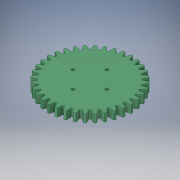
# Autodesk Inventor part: 000.302 - Втулка
Saved by Autodesk Inventor 2019 (Build 230136000, 136)
## iProperties
Created: 2020-02-27
Part Number: 000.302 - Втулка
Material: Пластик АБС
Document SubType Name: Modeling
Designer: Петров Иван
Density: 1.06 g/cm^3
Appearance: Гладкий — темный цвет морской волны
Author: Петров Иван
Autodesk Inventor part; units mm, degrees
ref_plane "YZ Plane" through (0, 0, 0) normal (1, 0, 0) x (0, 1, 0)
ref_plane "XZ Plane" through (0, 0, 0) normal (0, 1, 0) x (-1, 0, 0)
ref_plane "XY Plane" through (0, 0, 0) normal (0, 0, 1) x (1, 0, 0)
sketch "Эскиз1" plane through (0, 0, 0) normal (0, 1, 0) x (-1, 0, 0)
  circle A0 centre (0, 0) radius 12.5
  dimension "d0" = 25
  constraints: 1 centre point, 1 coincident
  measures "d0" diameter of A0
extrude "Выдавливание1" add sketch "Эскиз1" along normal blind 8
sketch "Эскиз2" plane through (0, 8, 0) normal (0, 1, 0) x (1, 0, 0)
  circle A0 centre (0, 0) radius 23
  dimension "d3" = 46
  constraints: 1 centre point, 1 coincident
  measures "d3" diameter of A0
extrude "Выдавливание2" add sketch "Эскиз2" along normal blind 2
sketch "Эскиз3" plane through (0, 10, 0) normal (0, 1, 0) x (1, 0, 0)
  arc A0 (-8.1938, 41.193) -> (-8.7829, 35.8928) centre (15.46, 35.881) ccw
  arc A1 (-8.7829, 35.8928) -> (-10.3402, 35.4755) centre (0, 0) ccw
  arc A2 (-10.3402, 35.4755) -> (-13.5005, 39.7711) centre (-31.3293, 23.3439) ccw
  arc A3 (-13.5005, 39.7711) -> (-15.2224, 39.1443) centre (0, 0) ccw
  arc A4 (-15.2224, 39.1443) -> (-14.8822, 33.8224) centre (8.9945, 38.0205) ccw
  arc A5 (-14.8822, 33.8224) -> (-16.3433, 33.141) centre (0, 0) ccw
  arc A6 (-16.3433, 33.141) -> (-20.2015, 36.8225) centre (-34.9069, 17.549) ccw
  arc A7 (-20.2015, 36.8225) -> (-21.7885, 35.9063) centre (0, 0) ccw
  arc A8 (-21.7885, 35.9063) -> (-20.5293, 30.7243) centre (2.2556, 39.0048) ccw
  arc A9 (-20.5293, 30.7243) -> (-21.8499, 29.7995) centre (0, 0) ccw
  arc A10 (-21.8499, 29.7995) -> (-26.2888, 32.7551) centre (-37.424, 11.2208) ccw
  arc A11 (-26.2888, 32.7551) -> (-27.6925, 31.5773) centre (0, 0) ccw
  arc A12 (-27.6925, 31.5773) -> (-25.5526, 26.6926) centre (-4.5518, 38.8039) ccw
  arc A13 (-25.5526, 26.6926) -> (-26.6926, 25.5526) centre (0, 0) ccw
  arc A14 (-26.6926, 25.5526) -> (-31.5773, 27.6925) centre (-38.8039, 4.5518) ccw
  arc A15 (-31.5773, 27.6925) -> (-32.7551, 26.2888) centre (0, 0) ccw
  arc A16 (-32.7551, 26.2888) -> (-29.7995, 21.8499) centre (-11.2208, 37.424) ccw
  arc A17 (-29.7995, 21.8499) -> (-30.7243, 20.5293) centre (0, 0) ccw
  arc A18 (-30.7243, 20.5293) -> (-35.9063, 21.7885) centre (-39.0048, -2.2556) ccw
  arc A19 (-35.9063, 21.7885) -> (-36.8225, 20.2015) centre (0, 0) ccw
  arc A20 (-36.8225, 20.2015) -> (-33.141, 16.3433) centre (-17.549, 34.9069) ccw
  arc A21 (-33.141, 16.3433) -> (-33.8224, 14.8822) centre (0, 0) ccw
  arc A22 (-33.8224, 14.8822) -> (-39.1443, 15.2224) centre (-38.0205, -8.9945) ccw
  arc A23 (-39.1443, 15.2224) -> (-39.7711, 13.5005) centre (0, 0) ccw
  arc A24 (-39.7711, 13.5005) -> (-35.4755, 10.3402) centre (-23.3439, 31.3293) ccw
  arc A25 (-35.4755, 10.3402) -> (-35.8928, 8.7829) centre (0, 0) ccw
  arc A26 (-35.8928, 8.7829) -> (-41.193, 8.1938) centre (-35.881, -15.46) ccw
  arc A27 (-41.193, 8.1938) -> (-41.5112, 6.3892) centre (0, 0) ccw
  arc A28 (-41.5112, 6.3892) -> (-36.7321, 4.0228) centre (-28.4295, 26.7997) ccw
  arc A29 (-36.7321, 4.0228) -> (-36.8726, 2.4168) centre (0, 0) ccw
  arc A30 (-36.8726, 2.4168) -> (-41.99, 0.9162) centre (-32.6513, -21.4558) ccw
  arc A31 (-41.99, 0.9162) -> (-41.99, -0.9162) centre (0, 0) ccw
  arc A32 (-41.99, -0.9162) -> (-36.8726, -2.4168) centre (-32.6513, 21.4558) ccw
  arc A33 (-36.8726, -2.4168) -> (-36.7321, -4.0228) centre (0, 0) ccw
  arc A34 (-36.7321, -4.0228) -> (-41.5112, -6.3892) centre (-28.4295, -26.7997) ccw
  arc A35 (-41.5112, -6.3892) -> (-41.193, -8.1938) centre (0, 0) ccw
  arc A36 (-41.193, -8.1938) -> (-35.8928, -8.7829) centre (-35.881, 15.46) ccw
  arc A37 (-35.8928, -8.7829) -> (-35.4755, -10.3402) centre (0, 0) ccw
  arc A38 (-35.4755, -10.3402) -> (-39.7711, -13.5005) centre (-23.3439, -31.3293) ccw
  arc A39 (-39.7711, -13.5005) -> (-39.1443, -15.2224) centre (0, 0) ccw
  arc A40 (-39.1443, -15.2224) -> (-33.8224, -14.8822) centre (-38.0205, 8.9945) ccw
  arc A41 (-33.8224, -14.8822) -> (-33.141, -16.3433) centre (0, 0) ccw
  arc A42 (-33.141, -16.3433) -> (-36.8225, -20.2015) centre (-17.549, -34.9069) ccw
  arc A43 (-36.8225, -20.2015) -> (-35.9063, -21.7885) centre (0, 0) ccw
  arc A44 (-35.9063, -21.7885) -> (-30.7243, -20.5293) centre (-39.0048, 2.2556) ccw
  arc A45 (-30.7243, -20.5293) -> (-29.7995, -21.8499) centre (0, 0) ccw
  arc A46 (-29.7995, -21.8499) -> (-32.7551, -26.2888) centre (-11.2208, -37.424) ccw
  arc A47 (-32.7551, -26.2888) -> (-31.5773, -27.6925) centre (0, 0) ccw
  arc A48 (-31.5773, -27.6925) -> (-26.6926, -25.5526) centre (-38.8039, -4.5518) ccw
  arc A49 (-26.6926, -25.5526) -> (-25.5526, -26.6926) centre (0, 0) ccw
  arc A50 (-25.5526, -26.6926) -> (-27.6925, -31.5773) centre (-4.5518, -38.8039) ccw
  arc A51 (-27.6925, -31.5773) -> (-26.2888, -32.7551) centre (0, 0) ccw
  arc A52 (-26.2888, -32.7551) -> (-21.8499, -29.7995) centre (-37.424, -11.2208) ccw
  arc A53 (-21.8499, -29.7995) -> (-20.5293, -30.7243) centre (0, 0) ccw
  arc A54 (-20.5293, -30.7243) -> (-21.7885, -35.9063) centre (2.2556, -39.0048) ccw
  arc A55 (-21.7885, -35.9063) -> (-20.2015, -36.8225) centre (0, 0) ccw
  arc A56 (-20.2015, -36.8225) -> (-16.3433, -33.141) centre (-34.9069, -17.549) ccw
  arc A57 (-16.3433, -33.141) -> (-14.8822, -33.8224) centre (0, 0) ccw
  arc A58 (-14.8822, -33.8224) -> (-15.2224, -39.1443) centre (8.9945, -38.0205) ccw
  arc A59 (-15.2224, -39.1443) -> (-13.5005, -39.7711) centre (0, 0) ccw
  arc A60 (-13.5005, -39.7711) -> (-10.3402, -35.4755) centre (-31.3293, -23.3439) ccw
  arc A61 (-10.3402, -35.4755) -> (-8.7829, -35.8928) centre (0, 0) ccw
  arc A62 (-8.7829, -35.8928) -> (-8.1938, -41.193) centre (15.46, -35.881) ccw
  arc A63 (-8.1938, -41.193) -> (-6.3892, -41.5112) centre (0, 0) ccw
  arc A64 (-6.3892, -41.5112) -> (-4.0228, -36.7321) centre (-26.7997, -28.4295) ccw
  arc A65 (-4.0228, -36.7321) -> (-2.4168, -36.8726) centre (0, 0) ccw
  arc A66 (-2.4168, -36.8726) -> (-0.9162, -41.99) centre (21.4558, -32.6513) ccw
  arc A67 (-0.9162, -41.99) -> (0.9162, -41.99) centre (0, 0) ccw
  arc A68 (0.9162, -41.99) -> (2.4168, -36.8726) centre (-21.4558, -32.6513) ccw
  arc A69 (2.4168, -36.8726) -> (4.0228, -36.7321) centre (0, 0) ccw
  arc A70 (4.0228, -36.7321) -> (6.3892, -41.5112) centre (26.7997, -28.4295) ccw
  arc A71 (6.3892, -41.5112) -> (8.1938, -41.193) centre (0, 0) ccw
  arc A72 (8.1938, -41.193) -> (8.7829, -35.8928) centre (-15.46, -35.881) ccw
  arc A73 (8.7829, -35.8928) -> (10.3402, -35.4755) centre (0, 0) ccw
  arc A74 (10.3402, -35.4755) -> (13.5005, -39.7711) centre (31.3293, -23.3439) ccw
  arc A75 (13.5005, -39.7711) -> (15.2224, -39.1443) centre (0, 0) ccw
  arc A76 (15.2224, -39.1443) -> (14.8822, -33.8224) centre (-8.9945, -38.0205) ccw
  arc A77 (14.8822, -33.8224) -> (16.3433, -33.141) centre (0, 0) ccw
  arc A78 (16.3433, -33.141) -> (20.2015, -36.8225) centre (34.9069, -17.549) ccw
  arc A79 (20.2015, -36.8225) -> (21.7885, -35.9063) centre (0, 0) ccw
  arc A80 (21.7885, -35.9063) -> (20.5293, -30.7243) centre (-2.2556, -39.0048) ccw
  arc A81 (20.5293, -30.7243) -> (21.8499, -29.7995) centre (0, 0) ccw
  arc A82 (21.8499, -29.7995) -> (26.2888, -32.7551) centre (37.424, -11.2208) ccw
  arc A83 (26.2888, -32.7551) -> (27.6925, -31.5773) centre (0, 0) ccw
  arc A84 (27.6925, -31.5773) -> (25.5526, -26.6926) centre (4.5518, -38.8039) ccw
  arc A85 (25.5526, -26.6926) -> (26.6926, -25.5526) centre (0, 0) ccw
  arc A86 (26.6926, -25.5526) -> (31.5773, -27.6925) centre (38.8039, -4.5518) ccw
  arc A87 (31.5773, -27.6925) -> (32.7551, -26.2888) centre (0, 0) ccw
  arc A88 (32.7551, -26.2888) -> (29.7995, -21.8499) centre (11.2208, -37.424) ccw
  arc A89 (29.7995, -21.8499) -> (30.7243, -20.5293) centre (0, 0) ccw
  arc A90 (30.7243, -20.5293) -> (35.9063, -21.7885) centre (39.0048, 2.2556) ccw
  arc A91 (35.9063, -21.7885) -> (36.8225, -20.2015) centre (0, 0) ccw
  arc A92 (36.8225, -20.2015) -> (33.141, -16.3433) centre (17.549, -34.9069) ccw
  arc A93 (33.141, -16.3433) -> (33.8224, -14.8822) centre (0, 0) ccw
  arc A94 (33.8224, -14.8822) -> (39.1443, -15.2224) centre (38.0205, 8.9945) ccw
  arc A95 (39.1443, -15.2224) -> (39.7711, -13.5005) centre (0, 0) ccw
  arc A96 (39.7711, -13.5005) -> (35.4755, -10.3402) centre (23.3439, -31.3293) ccw
  arc A97 (35.4755, -10.3402) -> (35.8928, -8.7829) centre (0, 0) ccw
  arc A98 (35.8928, -8.7829) -> (41.193, -8.1938) centre (35.881, 15.46) ccw
  arc A99 (41.193, -8.1938) -> (41.5112, -6.3892) centre (0, 0) ccw
  arc A100 (41.5112, -6.3892) -> (36.7321, -4.0228) centre (28.4295, -26.7997) ccw
  arc A101 (36.7321, -4.0228) -> (36.8726, -2.4168) centre (0, 0) ccw
  arc A102 (36.8726, -2.4168) -> (41.99, -0.9162) centre (32.6513, 21.4558) ccw
  arc A103 (41.99, -0.9162) -> (41.99, 0.9162) centre (0, 0) ccw
  arc A104 (41.99, 0.9162) -> (36.8726, 2.4168) centre (32.6513, -21.4558) ccw
  arc A105 (36.8726, 2.4168) -> (36.7321, 4.0228) centre (0, 0) ccw
  arc A106 (36.7321, 4.0228) -> (41.5112, 6.3892) centre (28.4295, 26.7997) ccw
  arc A107 (41.5112, 6.3892) -> (41.193, 8.1938) centre (0, 0) ccw
  arc A108 (41.193, 8.1938) -> (35.8928, 8.7829) centre (35.881, -15.46) ccw
  arc A109 (35.8928, 8.7829) -> (35.4755, 10.3402) centre (0, 0) ccw
  arc A110 (35.4755, 10.3402) -> (39.7711, 13.5005) centre (23.3439, 31.3293) ccw
  arc A111 (39.7711, 13.5005) -> (39.1443, 15.2224) centre (0, 0) ccw
  arc A112 (39.1443, 15.2224) -> (33.8224, 14.8822) centre (38.0205, -8.9945) ccw
  arc A113 (33.8224, 14.8822) -> (33.141, 16.3433) centre (0, 0) ccw
  arc A114 (33.141, 16.3433) -> (36.8225, 20.2015) centre (17.549, 34.9069) ccw
  arc A115 (36.8225, 20.2015) -> (35.9063, 21.7885) centre (0, 0) ccw
  arc A116 (35.9063, 21.7885) -> (30.7243, 20.5293) centre (39.0048, -2.2556) ccw
  arc A117 (30.7243, 20.5293) -> (29.7995, 21.8499) centre (0, 0) ccw
  arc A118 (29.7995, 21.8499) -> (32.7551, 26.2888) centre (11.2208, 37.424) ccw
  arc A119 (32.7551, 26.2888) -> (31.5773, 27.6925) centre (0, 0) ccw
  arc A120 (31.5773, 27.6925) -> (26.6926, 25.5526) centre (38.8039, 4.5518) ccw
  arc A121 (26.6926, 25.5526) -> (25.5526, 26.6926) centre (0, 0) ccw
  arc A122 (25.5526, 26.6926) -> (27.6925, 31.5773) centre (4.5518, 38.8039) ccw
  arc A123 (27.6925, 31.5773) -> (26.2888, 32.7551) centre (0, 0) ccw
  arc A124 (26.2888, 32.7551) -> (21.8499, 29.7995) centre (37.424, 11.2208) ccw
  arc A125 (21.8499, 29.7995) -> (20.5293, 30.7243) centre (0, 0) ccw
  arc A126 (20.5293, 30.7243) -> (21.7885, 35.9063) centre (-2.2556, 39.0048) ccw
  arc A127 (21.7885, 35.9063) -> (20.2015, 36.8225) centre (0, 0) ccw
  arc A128 (20.2015, 36.8225) -> (16.3433, 33.141) centre (34.9069, 17.549) ccw
  arc A129 (16.3433, 33.141) -> (14.8822, 33.8224) centre (0, 0) ccw
  arc A130 (14.8822, 33.8224) -> (15.2224, 39.1443) centre (-8.9945, 38.0205) ccw
  arc A131 (15.2224, 39.1443) -> (13.5005, 39.7711) centre (0, 0) ccw
  arc A132 (13.5005, 39.7711) -> (10.3402, 35.4755) centre (31.3293, 23.3439) ccw
  arc A133 (10.3402, 35.4755) -> (8.7829, 35.8928) centre (0, 0) ccw
  arc A134 (8.7829, 35.8928) -> (8.1938, 41.193) centre (-15.46, 35.881) ccw
  arc A135 (8.1938, 41.193) -> (6.3892, 41.5112) centre (0, 0) ccw
  arc A136 (6.3892, 41.5112) -> (4.0228, 36.7321) centre (26.7997, 28.4295) ccw
  arc A137 (4.0228, 36.7321) -> (2.4168, 36.8726) centre (0, 0) ccw
  arc A138 (2.4168, 36.8726) -> (0.9162, 41.99) centre (-21.4558, 32.6513) ccw
  arc A139 (0.9162, 41.99) -> (-0.9162, 41.99) centre (0, 0) ccw
  arc A140 (-0.9162, 41.99) -> (-2.4168, 36.8726) centre (21.4558, 32.6513) ccw
  arc A141 (-2.4168, 36.8726) -> (-4.0228, 36.7321) centre (0, 0) ccw
  arc A142 (-4.0228, 36.7321) -> (-6.3892, 41.5112) centre (-26.7997, 28.4295) ccw
  arc A143 (-6.3892, 41.5112) -> (-8.1938, 41.193) centre (0, 0) ccw
  constraints: 288 point on circle, 144 centre point
extrude "Выдавливание3" add sketch "Эскиз3" along normal blind 8
sketch "Эскиз4" plane through (0, 8, 0) normal (0, -1, 0) x (1, 0, 0)
  line L0 (0, 0) -> (0, -17)
  line L1 (4, -17) -> (2, -20.4641)
  line L2 (2, -20.4641) -> (-2, -20.4641)
  line L3 (-2, -20.4641) -> (-4, -17)
  line L4 (-4, -17) -> (-2, -13.5359)
  line L5 (-2, -13.5359) -> (2, -13.5359)
  line L6 (2, -13.5359) -> (4, -17)
  dimension "d8" = 17
  dimension "d9" = 8
  constraints: 14 end point, 1 coincident, 1 vertical, 13 other
  measures "d8" distance of L0.start L0.end
  measures "d9" distance of L3.end L1.start
extrude "Выдавливание4" cut sketch "Эскиз4" against normal blind 3.3
sketch "Эскиз6" plane through (0, 11.3, 0) normal (0, -1, 0) x (1, 0, 0)
  circle A0 centre (0, 0) radius 12.5 projected
  line L0 (0, 0) -> (0, -17)
  line L1 (3.05, -17) -> (1.525, -19.6414)
  line L2 (1.525, -19.6414) -> (-1.525, -19.6414)
  line L3 (-1.525, -19.6414) -> (-3.05, -17)
  line L4 (-3.05, -17) -> (-1.525, -14.3586)
  line L5 (-1.525, -14.3586) -> (1.525, -14.3586)
  line L6 (1.525, -14.3586) -> (3.05, -17)
  dimension "d16" = 17
  dimension "d17" = 6.1
  constraints: 14 end point, 1 coincident, 1 vertical, 13 other
  measures "d16" distance of L0.start L0.end
  measures "d17" distance of L3.end L1.start
extrude "Выдавливание6" cut sketch "Эскиз6" against normal blind 2.6 contours L1 L2 L3 L4 L5 L6
sketch "Эскиз7" plane through (0, 13.9, 0) normal (0, -1, 0) x (1, 0, 0)
  circle A0 centre (0, 0) radius 12.5 projected
  line L0 (0, 0) -> (0, -17)
  circle A1 centre (0, -17) radius 1.5
  dimension "d20" = 17
  dimension "d21" = 3
  constraints: 2 end point, 1 centre point, 1 coincident, 1 vertical
  measures "d20" distance of L0.start L0.end
  measures "d21" diameter of A1
extrude "Выдавливание7" cut sketch "Эскиз7" against normal through all contours A1
pattern_circular "Круговой массив1" count 4 over 360 about axis through (0, 0, 0) along (0, 1, 0) of "Выдавливание6", "Выдавливание7", "Выдавливание4"
